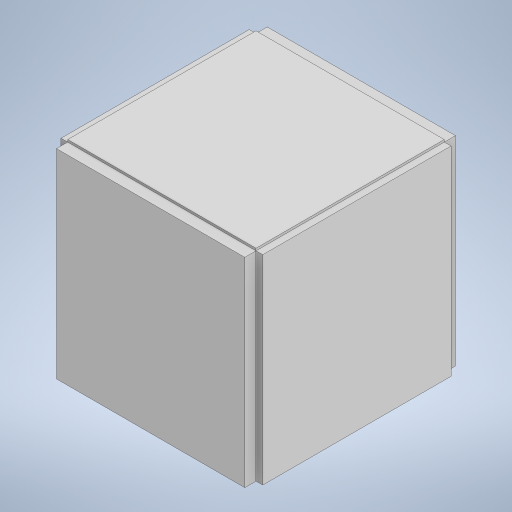
# Autodesk Inventor part: Payload
Saved by Autodesk Inventor 2023 (Build 270158000, 158)
## iProperties
Created: 2022-08-05
Part Number: Payload
Material: Generic
Document SubType Name: Modeling
Designer: Aditya Bansal
Density: 1 g/cm^3
Appearance: Default
Author: Aditya Bansal
Autodesk Inventor part; units mm, degrees
ref_plane "YZ Plane" through (0, 0, 0) normal (1, 0, 0) x (0, 1, 0)
ref_plane "XZ Plane" through (0, 0, 0) normal (0, 1, 0) x (-1, 0, 0)
ref_plane "XY Plane" through (0, 0, 0) normal (0, 0, 1) x (1, 0, 0)
sketch "Sketch1" plane through (0, 0, 0) normal (0, 1, 0) x (-1, 0, 0)
  line L0 (0, 0) -> (-90, 0)
  line L1 (-90, 0) -> (-90, -94)
  line L2 (-90, -94) -> (0, -94)
  line L3 (0, -94) -> (0, 0)
  line L4 (0, -94) -> (-3, -94)
  line L5 (-3, -94) -> (-3, -89)
  line L6 (-3, -89) -> (0, -89)
  line L7 (0, -89) -> (0, -94)
  line L8 (-90, -94) -> (-87, -94)
  line L9 (-87, -94) -> (-87, -89)
  line L10 (-87, -89) -> (-90, -89)
  line L11 (-90, -89) -> (-90, -94)
  line L12 (0, 0) -> (-3, 0)
  line L13 (-3, 0) -> (-3, -5)
  line L14 (-3, -5) -> (0, -5)
  line L15 (0, -5) -> (0, 0)
  line L16 (-90, 0) -> (-87, 0)
  line L17 (-87, 0) -> (-87, -5)
  line L18 (-87, -5) -> (-90, -5)
  line L19 (-90, -5) -> (-90, 0)
  dimension "d0" = 94
  dimension "d1" = 90
  dimension "d2" = 5
  dimension "d3" = 3
  constraints: 40 end point, 10 parallel, 6 equal length, 5 horizontal, 5 perpendicular
  measures "d0" distance of L0.end L1.end
  measures "d1" distance of L1.end L2.end
  measures "d2" distance of L16.end L17.end
  measures "d3" distance of L13.end L14.end
extrude "Extrusion1" add sketch "Sketch1" along normal blind 89 contours L13 L14 L3 L6 L5 L2 L9 L10 L1 L18 L17 L0
sketch "Sketch3" plane through (0, 89, 0) normal (0, 1, 0) x (1, 0, 0)
  line L0 (3, 94) -> (3, 89) projected
  line L1 (87, 5) -> (3, 5)
  line L2 (3, 5) -> (3, 89)
  line L3 (3, 89) -> (87, 89)
  line L4 (87, 89) -> (87, 5)
  point P0 (0, 0)
  constraints: 8 end point, 2 parallel, 1 horizontal, 1 perpendicular
extrude "Extrusion2" add sketch "Sketch3" along normal blind 1
body "Solid1"
